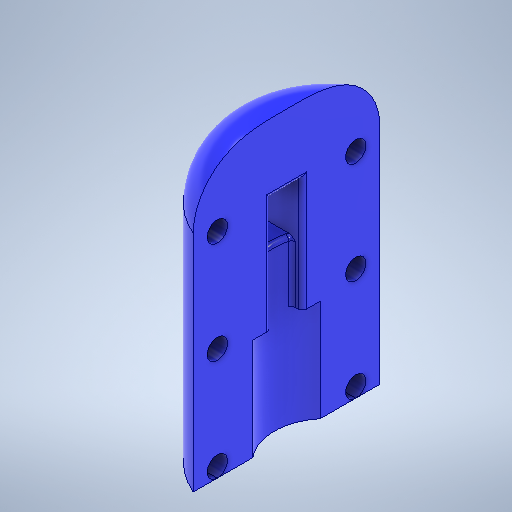
# Autodesk Inventor part: Switch Side
Saved by Autodesk Inventor 2025.2 (Build 292293000, 293)
## iProperties
Created: 2025-02-16
Part Number: Switch Side
Material: Generic
Document SubType Name: Modeling
Designer: eason
Density: 1 g/cm^3
Appearance: Blue - Wall Paint - Glossy
Author: eason
Autodesk Inventor part; units mm, degrees
sketch "Sketch1" plane through (0, 0, 0) normal (0, 0, 1) x (1, 0, 0)
  line L0 (0, 0) -> (0, 70)
  line L1 (0, 0) -> (25, 0)
  line L2 (25, 0) -> (25, 55)
  line L3 (0, -14.6213) -> (0, 87.7279) projected
  line L4 (0, 70) -> (10, 70)
  arc A0 (25, 55) -> (10, 70) centre (10, 55) ccw
  dimension "d0" = 70
  dimension "d1" = 25
  dimension "d2" = 10
  constraints: 8 end point, 2 point on circle, 2 tangent, 2 vertical, 1 centre point, 1 horizontal, 1 perpendicular
  measures "d0" distance of L0.start L0.end
  measures "d1" distance of L0.start L1.end
  measures "d2" distance of L0.end L4.end
revolve "Revolution1" add sketch "Sketch1" angle 360 about axis through (0, -10, 0) along (0, 1, 0)
sketch "Sketch2" plane through (0, 0, 0) normal (0, -1, 0) x (1, 0, 0)
  circle A0 centre (0, 0) radius 10
  dimension "d4" = 20
  constraints: 1 centre point, 1 coincident
  measures "d4" diameter of A0
extrude "Extrusion1" cut sketch "Sketch2" against normal blind 25
sketch "Sketch3" plane through (0, 70, 0) normal (0, 1, 0) x (1, 0, 0)
  circle A0 centre (0, 0) radius 10 projected
  line L0 (10, 0) -> (-10, 0) construction
  line L1 (-35, 0) -> (35, 0) construction
  constraints: 2 end point, 2 point on circle, 1 collinear
ref_plane "Work Plane1" through (10, 70, 0) normal (1, 0, 0) x (0, 1, 0)
ref_plane "Work Plane2" through (-10, 70, 0) normal (1, 0, 0) x (0, 1, 0)
ref_plane "Work Plane3" through (0, 27.5, 25) normal (0, 0, 1) x (1, 0, 0)
sketch "Sketch4" plane through (0, 27.5, 25) normal (0, 0, 1) x (1, 0, 0)
  line L0 (-10, 56.5) -> (-10, -41.5) projected
  line L1 (10, 56.5) -> (10, -41.5) projected
  line L2 (25, -27.5) -> (-25, -27.5) projected
  line L3 (25, -27.5) -> (25, 27.5) projected
  arc A0 (25, 27.5) -> (10, 42.5) centre (10, 27.5) ccw projected
  line L4 (10, 42.5) -> (-10, 42.5) projected
  point P0 (0, -27.5)
  point P1 (-10, -27.5)
extrude "Extrusion2" cut sketch "Sketch4" against normal through all
sketch "Sketch5" plane through (-10, 0, 22.9129) normal (1, 0, 0) x (0, 0, -1)
  circle A0 centre (5.9129, 2.5) radius 2.5
  line L0 (45.8258, 0) -> (0, 0) projected
  line L1 (22.9129, -14.0011) -> (22.9129, 84.0066) projected
  circle A1 centre (39.9129, 2.5) radius 2.5
  circle A2 centre (5.9129, 27.5) radius 2.5
  circle A3 centre (39.9129, 27.5) radius 2.5
  circle A4 centre (5.9129, 52.5) radius 2.5
  circle A5 centre (39.9129, 52.5) radius 2.5
  point P0 (22.9129, 0)
  dimension "d10" = 5
  dimension "d11" = 17
  dimension "d14" = 34
  dimension "d17" = 25
  constraints: 6 centre point, 1 horizontal, 1 tangent, 1 vertical, 10 other
  measures "d10" diameter of A0
  measures "d11" distance from line of L1 A0.centre
  measures "d14" distance of A0.centre A1.centre
  measures "d17" distance of A0.centre A2.centre
extrude "Extrusion3" cut sketch "Sketch5" against normal blind 5
sketch "Sketch6" plane through (-10, 0, 22.9129) normal (1, 0, 0) x (0, 0, -1)
  line L0 (19.0129, 53.2) -> (26.8129, 53.2)
  line L1 (26.8129, 53.2) -> (26.8129, 40)
  line L2 (26.8129, 40) -> (19.0129, 40)
  line L3 (19.0129, 40) -> (19.0129, 53.2)
  line L4 (22.9129, -14.0011) -> (22.9129, 84.0066) projected
  line L5 (39.9129, 0) -> (5.9129, 0) projected
  point P0 (22.9129, 0)
  point P1 (22.9129, 53.2)
  dimension "d22" = 7.8
  dimension "d23" = 13.2
  dimension "d24" = 40
  constraints: 8 end point, 2 parallel, 1 horizontal, 1 midpoint, 1 perpendicular, 1 point on line
  measures "d22" distance between parallel lines of L1 L3
  measures "d23" distance between parallel lines of L2 L0
  measures "d24" distance between parallel lines of L5 L2
extrude "Extrusion4" cut sketch "Sketch6" against normal blind 14
sketch "Sketch7" plane through (-24, 0, 22.9129) normal (1, 0, 0) x (0, 0, -1)
  line L0 (26.8129, 40) -> (19.0129, 40) projected
  line L1 (19.0129, 53.2) -> (26.8129, 40) construction
  line L2 (19.0129, 53.2) -> (26.8129, 53.2) projected
  line L3 (26.8129, 53.2) -> (19.0129, 40) construction
  circle A0 centre (22.9129, 46.6) radius 3
  point P0 (22.9129, 0)
  dimension "d27" = 6
  constraints: 4 end point, 1 centre point, 1 midpoint
  measures "d27" diameter of A0
extrude "Extrusion5" cut sketch "Sketch7" against normal through all
sketch "Sketch8" plane through (0, 0, 0) normal (0, -1, 0) x (1, 0, 0)
  circle A0 centre (0, 0) radius 13
  dimension "d30" = 26
  constraints: 1 centre point, 1 coincident
  measures "d30" diameter of A0
extrude "Extrusion6" cut sketch "Sketch8" against normal blind 25
sketch "Sketch9" plane through (-10, 0, -22.9129) normal (1, 0, 0) x (0, 0, -1)
  line L0 (-19.0129, 40) -> (-26.8129, 40) projected
  line L1 (-31.2195, 25) -> (-14.6063, 25) projected
  line L2 (-26.8129, 40) -> (-19.0129, 40)
  line L3 (-19.0129, 40) -> (-19.0129, 25)
  line L4 (-19.0129, 25) -> (-26.8129, 25)
  line L5 (-26.8129, 25) -> (-26.8129, 40)
  line L6 (-19.0129, 53.2) -> (-19.0129, 40) projected
  point P0 (-22.9129, 0)
  constraints: 8 end point, 2 parallel, 1 collinear, 1 horizontal, 1 perpendicular, 1 point on line
extrude "Extrusion7" cut sketch "Sketch9" against normal up to surface round surface about axis through (0, 0, 0) along (0, 1, 0) radius 13 far side no
fillet "Fillet1" radius 1 6 edges at (-12.4012, 32.5, -3.9) (-12.4012, 32.5, 3.9) (-13, 40, 0) (-10, 39.1, -3.9) (-10, 39.1, 3.9) (-10, 53.2, 0)
body "Solid1"
